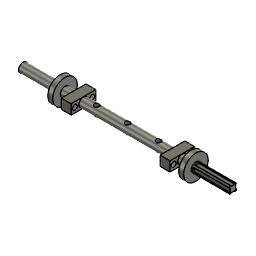
Dribbler Rod (Autodesk Fusion 360 design; units mm, degrees)
part number: 2026-04-20-21-14-20-702
Autodesk Fusion 360 part; units mm, degrees
sketch "Sketch1" plane through (0, 0, 0) normal (1, 0, 0) x (0, 0, -1)
  circle A0 centre (0, 0) radius 1.9
  dimension "d1" = 3.8
  constraint coincident A0.centre origin
  measures "d1" diameter of A0
extrude "Extrude1" add sketch "Sketch1" along normal blind 65
extrude "Extrude2" add 1 faces at (65, -0.5093, -0.5831) along direction (1, 0, 0) blind 10
sketch "Sketch2" plane through (0, 0, 0) normal (0, 1, 0) x (1, 0, 0)
  line L0 (0, 0) -> (37.5, 0)
  circle A0 centre (37.5, 0) radius 1
  line L1 (0, 0) -> (25, 0)
  circle A1 centre (25, 0) radius 1
  line L2 (37.5, 0) -> (50, 0)
  circle A2 centre (50, 0) radius 1
  dimension "d6" = 37.5
  dimension "d7" = 2
  dimension "d8" = 25
  dimension "d9" = 2
  dimension "d10" = 12.5
  dimension "d11" = 2
  constraint coincident L0.start L1.start
  constraint horizontal L0
  constraint coincident L0.end A0.centre
  constraint parallel L0 L1
  constraint coincident L1.end A1.centre
  constraint parallel L0 L2
  constraint coincident L2.end A2.centre
  measures "d6" distance of L0.start L0.end
  measures "d7" diameter of A0
  measures "d8" distance of L0.start L1.end
  measures "d9" diameter of A1
  measures "d10" distance of L0.end L2.end
  measures "d11" diameter of A2
extrude "Extrude3" cut sketch "Sketch2" along normal blind 3 and the other way blind 3
sketch "Sketch3" plane through (0, 0, 0) normal (0, 1, 0) x (1, 0, 0)
  line L0 (12.9545, 0) -> (60.4545, 0)
  line L1 (12.9545, 0) -> (17.9545, 0)
  line L2 (0, 0) -> (75, 0)
  line L3 (10, 0) -> (65, 0)
  line L4 (17.5, 0) -> (57.5, 0)
  line L5 (19.5, 5) -> (15.5, 5)
  line L6 (15.5, 5) -> (15.5, -5)
  line L7 (15.5, -5) -> (19.5, -5)
  line L8 (19.5, -5) -> (19.5, 5)
  line L9 (19.5, 5) -> (15.5, -5) construction
  line L10 (15.5, 5) -> (19.5, -5) construction
  line L11 (59.5, 5) -> (55.5, 5)
  line L12 (55.5, 5) -> (55.5, -5)
  line L13 (55.5, -5) -> (59.5, -5)
  line L14 (59.5, -5) -> (59.5, 5)
  line L15 (59.5, 5) -> (55.5, -5) construction
  line L16 (55.5, 5) -> (59.5, -5) construction
  point P0 (37.5, 0)
  point P1 (37.5, 0)
  point P2 (17.5, 0)
  point P3 (57.5, 0)
  dimension "d36" = 75
  dimension "d37" = 55
  dimension "d38" = 40
  dimension "d39" = 4
  dimension "d40" = 10
  dimension "d41" = 4
  dimension "d42" = 10
  constraint parallel L0 L1
  constraint coincident L2.start origin
  constraint horizontal L2
  constraint midpoint L3 P1
  constraint coincident L2 P1
  constraint parallel L2 L3
  constraint midpoint L4 P1
  constraint coincident P1 P0
  constraint coincident L0 P3
  constraint horizontal L5
  constraint perpendicular L5 L6
  constraint parallel L5 L7
  constraint parallel L6 L8
  constraint coincident L9 P2
  constraint coincident L10 P2
  constraint coincident P2 L4.start
  constraint horizontal L11
  constraint perpendicular L11 L12
  constraint parallel L11 L13
  constraint parallel L12 L14
  constraint coincident L15 P3
  constraint coincident L16 P3
  constraint coincident P3 L4.end
  measures "d36" distance of L2.start L2.end
  measures "d37" distance of L3.start L3.end
  measures "d38" distance of P2 P3
  measures "d39" distance of L6.end L7.end
  measures "d40" distance of L5.end L6.end
  measures "d41" distance of L12.end L13.end
  measures "d42" distance of L11.end L12.end
extrude "Extrude4" add sketch "Sketch3" along normal blind 2 and the other way blind 2
extrude "Extrude7" add sketch "Sketch3" along normal blind 2 and the other way blind 2
sketch "Sketch6" plane through (0, 0, 0) normal (-1, 0, 0) x (0, 0, 1)
  circle A0 centre (0, 0) radius 1.9
  line L0 (0, 0) -> (-3.5, 0)
  circle A1 centre (-3.5, 0) radius 1
  line L1 (0, 0) -> (3.5, 0)
  circle A2 centre (3.5, 0) radius 1
  dimension "d47" = 3.5
  dimension "d48" = 2
  dimension "d49" = 3.5
  dimension "d50" = 2
  constraint coincident A0.centre L0.start
  constraint horizontal L0
  constraint coincident L0.end A1.centre
  constraint parallel L0 L1
  constraint coincident L1.end A2.centre
  measures "d47" distance of A0.centre L0.end
  measures "d48" diameter of A1
  measures "d49" distance of A0.centre L1.end
  measures "d50" diameter of A2
extrude "Extrude8" cut sketch "Sketch6" against normal blind 75 contours A1 | A2
sketch "Sketch7" plane through (0, 0, 0) normal (0, 1, 0) x (1, 0, 0)
  line L0 (0, 0) -> (37.5, 0) construction
  line L1 (10, 0) -> (65, 0) construction
  line L2 (10, 0) -> (11, 0) construction
  line L3 (12, 5) -> (10, 5)
  line L4 (10, 5) -> (10, -5)
  line L5 (10, -5) -> (12, -5)
  line L6 (12, -5) -> (12, 5)
  line L7 (12, 5) -> (10, -5) construction
  line L8 (10, 5) -> (12, -5) construction
  line L9 (10, -1.9) -> (10, 1.9)
  line L10 (10, -1.9) -> (12, -1.9)
  line L11 (10, 1.9) -> (12, 1.9)
  line L12 (37.5, 0) -> (37.5, -5.856) construction
  line L13 (65, 5) -> (65, -5)
  line L14 (65, -5) -> (63, -5)
  line L15 (63, -5) -> (63, 5)
  line L16 (65, -1.9) -> (63, -1.9)
  line L17 (65, 1.9) -> (63, 1.9)
  line L18 (63, 5) -> (65, 5)
  point P0 (11, 0)
  dimension "d53" = 37.5
  dimension "d54" = 55
  dimension "d55" = 1
  dimension "d56" = 2
  dimension "d57" = 10
  dimension "d60" = 3.8
  constraint coincident L0.start origin
  constraint horizontal L0
  constraint midpoint L0.end L1
  constraint parallel L0 L1
  constraint parallel L0 L2
  constraint horizontal L3
  constraint perpendicular L3 L4
  constraint parallel L3 L5
  constraint parallel L4 L6
  constraint coincident L7 P0
  constraint coincident L8 P0
  constraint coincident P0 L2.end
  constraint midpoint L1.start L9
  constraint perpendicular L2 L9
  constraint coincident L6 L10.end
  constraint perpendicular L6 L10
  constraint coincident L6 L11.end
  constraint perpendicular L6 L11
  constraint perpendicular L1 L12
  constraint symmetric L3.start L12 L15.end
  constraint symmetric L3.end L12 L13.start
  constraint symmetric L4.end L12 L13.end
  constraint symmetric L5.end L12 L14.end
  constraint symmetric L9.start L12 L16.start
  constraint symmetric L9.end L12 L17.start
  constraint symmetric L10.end L12 L16.end
  constraint symmetric L11.end L12 L17.end
  measures "d53" distance of L0.start L0.end
  measures "d54" distance of L1.start L1.end
  measures "d55" distance of L1.start P0
  measures "d56" distance of L4.end L5.end
  measures "d57" distance of L3.end L4.end
  measures "d60" distance of L9.start L9.end
revolve "Revolve1" add sketch "Sketch7" angle 180 about axis through (0, 0, 0) along (-1, 0, 0) contours L3 L4 L6 L11 | L4 L5 L6 L10 | L13 L15 L17 L18 | L13 L14 L15 L16
sketch "Sketch8" plane through (75, 0, 0) normal (1, 0, 0) x (0, 0, -1)
  circle A0 centre (0, 0) radius 1.9
  circle A1 centre (0, 0) radius 2
  line L0 (0, 0) -> (0, 2)
  line L1 (0, 0) -> (-0.9, 0)
  line L2 (-0.9, 0) -> (-0.9, 1.7861)
  line L3 (0, 0) -> (0.9, 0)
  line L4 (0.9, 0) -> (0.9, 1.7861)
  line L5 (0, 2) -> (0, 1.15)
  line L6 (0.9, 1.15) -> (-0.9, 1.15)
  line L7 (-1.15, 0.9) -> (-1.15, -0.9)
  line L8 (0, -0.9) -> (-1.7861, -0.9)
  line L9 (0, 0.9) -> (-1.7861, 0.9)
  line L10 (-0.9, -1.15) -> (0.9, -1.15)
  line L11 (0.9, 0) -> (0.9, -1.7861)
  line L12 (-0.9, 0) -> (-0.9, -1.7861)
  line L13 (1.15, -0.9) -> (1.15, 0.9)
  line L14 (0, 0.9) -> (1.7861, 0.9)
  line L15 (0, -0.9) -> (1.7861, -0.9)
  dimension "d62" = 4
  dimension "d63" = 0.9
  dimension "d64" = 0.9
  dimension "d65" = 0.85
  dimension "d67" = 360
  constraint concentric A0 A1
  constraint coincident A0.centre A1.centre
  constraint coincident A1 L0.end
  constraint vertical L0
  constraint perpendicular L0 L1
  constraint coincident A1 L2.end
  constraint perpendicular L1 L2
  constraint perpendicular L0 L3
  constraint coincident A1 L4.end
  constraint perpendicular L3 L4
  constraint parallel L0 L5
  constraint midpoint L5.end L6
  constraint coincident L2 L6.end
  constraint perpendicular L2 L6
  measures "d62" diameter of A1
  measures "d63" distance of A0.centre L1.end
  measures "d64" distance of A0.centre L3.end
  measures "d65" distance of L0.end L5.end
extrude "Extrude9" cut sketch "Sketch8" against normal blind 9.5 contours A0 L13 L14 L15 | A0 L0 L4 L5 L6 | A0 L10 L11 L12 | A0 L0 L2 L5 L6 | A0 L7 L8 L9
fillet "Fillet1" radius 0.1 8 edges at (70.25, 0.9, 1.15) (70.25, -0.9, 1.15) (70.25, 1.15, -0.9) (70.25, 1.15, 0.9) (70.25, 0.9, -1.15) (70.25, -0.9, -1.15) (70.25, -1.15, -0.9) (70.25, -1.15, 0.9)
fillet "Fillet2" radius 0.1 8 edges at (70.25, 0.9, 1.6733) (70.25, -0.9, 1.6733) (70.25, -1.6733, 0.9) (70.25, -1.6733, -0.9) (70.25, -0.9, -1.6733) (70.25, 0.9, -1.6733) (70.25, 1.6733, -0.9) (70.25, 1.6733, 0.9)
extrude "Extrude10" add 1 faces at (75, 0.2667, 0.3833) along direction (1, 0, 0) blind 5
extrude "Extrude11" add 1 faces at (0, -0.5093, -0.5831) along direction (-1, 0, 0) blind 5
equation "d6 = ( 75 / 2 ) * 1 mm"
